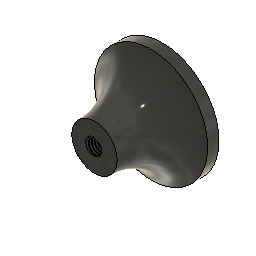
Pin_Release_Handle v3 (Autodesk Fusion 360 design; units mm, degrees)
Autodesk Fusion 360 part; units mm, degrees
sketch "Sketch1" plane through (0, 0, 0) normal (0, 0, 1) x (1, 0, 0)
  line L0 (0, 0) -> (4, 0)
  line L1 (4, 0) -> (4, 12) construction
  line L2 (4, 0) -> (10, 0) construction
  line L3 (10, 0) -> (10, 10) construction
  line L4 (10, 0) -> (4, 0) construction
  line L5 (10, 10) -> (10, 12)
  line L6 (0, 0) -> (0, 12)
  line L7 (0, 12) -> (10, 12)
  arc A0 (10, 10) -> (4, 0) centre (15.3333, 0) ccw
  dimension "d1" = 4
  dimension "d2" = 12
  dimension "d5" = 90
  dimension "d7" = 12
  dimension "d9" = 2
  dimension "d10" = 6
  constraint coincident L0.start L6.start
  constraint horizontal L0
  constraint perpendicular L0 L1
  constraint perpendicular L1 L2
  constraint coincident L2.end L3.start
  constraint parallel L3 L5
  constraint perpendicular L0 L6
  constraint horizontal L7
  constraint tangent L1 A0
  measures "d1" distance of L0.start L0.end
  measures "d2" distance of L0.end L1.end
  measures "d5" angle of L3 L4
  measures "d7" distance of L0.start L6.end
  measures "d9" distance of L3.end L5.end
  measures "d10" distance of L0.end L2.end
revolve "Revolve2" add sketch "Sketch1" angle 360 about axis through (0, 0, 0) along (0, 1, 0)
sketch "Sketch2" plane through (0, 0, 0) normal (0, -1, 0) x (1, 0, 0)
  circle A0 centre (0, 0) radius 4
  constraint coincident A0.centre origin
hole "Hole1" at (0, 0, 0) direction (0, 1, 0) diameter 2.529 depth 7 tip angle 180
thread "Thread1" "ISO Metric profile 3.0 M3x0.5 6H" major diameter 3.086 minor diameter 2.529 pitch 0.5 angle 60 modelled right hand crest width 0.1368 on face at (0.1259, 2.3333, -1.2582) crest through (0, 0.125, -1.2645)
